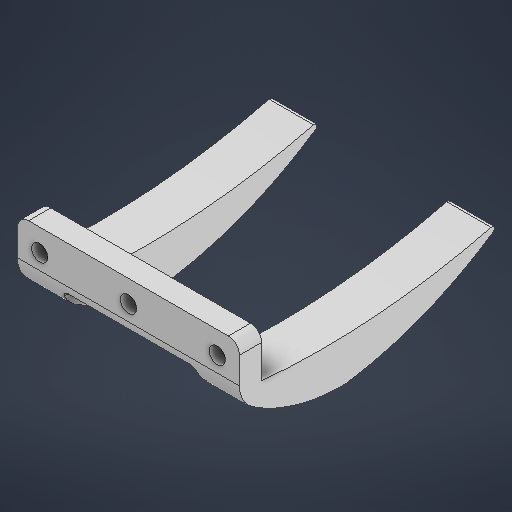
# Autodesk Inventor part: Second Stage Compression
Saved by Autodesk Inventor 2025 (Build 290162000, 162)
## iProperties
Created: 2024-12-29
Part Number: Second Stage Compression
Material: Generic
Document SubType Name: Modeling
Designer: Juan
Density: 1 g/cm^3
Appearance: Default
Author: Juan
Autodesk Inventor part; units mm, degrees
ref_plane "YZ Plane" through (0, 0, 0) normal (1, 0, 0) x (0, 1, 0)
ref_plane "XZ Plane" through (0, 0, 0) normal (0, 1, 0) x (-1, 0, 0)
ref_plane "XY Plane" through (0, 0, 0) normal (0, 0, 1) x (1, 0, 0)
sketch "Sketch1" plane through (0, 0, 0) normal (0, 0, 1) x (1, 0, 0)
  circle A0 centre (0, 0) radius 2.3241
  line L0 (0, 0) -> (12.7, 0)
  line L1 (12.7, 0) -> (25.4, 0)
  line L2 (0, 0) -> (-12.7, 0)
  line L3 (-12.7, 0) -> (-25.4, 0)
  circle A1 centre (-25.4, 0) radius 2.3241
  circle A2 centre (25.4, 0) radius 2.3241
  line L4 (-25.4, 0) -> (-31.75, 0)
  line L5 (25.4, 0) -> (31.75, 0)
  line L6 (-31.75, 6.35) -> (31.75, 6.35)
  line L7 (31.75, 6.35) -> (31.75, -6.35)
  line L8 (31.75, -6.35) -> (-31.75, -6.35)
  line L9 (-31.75, -6.35) -> (-31.75, 6.35)
  line L10 (-31.75, 6.35) -> (31.75, -6.35) construction
  line L11 (31.75, 6.35) -> (-31.75, -6.35) construction
  dimension "d0" = 4.6482
  dimension "d1" = 12.7
  dimension "d2" = 12.7
  dimension "d3" = 12.7
  dimension "d4" = 12.7
  dimension "d5" = 4.6482
  dimension "d6" = 4.6482
  dimension "d7" = 6.35
  dimension "d8" = 6.35
  dimension "d9" = 12.7
  constraints: 24 end point, 5 horizontal, 3 centre point, 3 coincident, 2 midpoint, 2 parallel, 2 point on line, 1 perpendicular
  measures "d0" diameter of A0
  measures "d1" distance of L0.start L0.end
  measures "d2" distance of L0.end L1.end
  measures "d3" distance of L0.start L2.end
  measures "d4" distance of L2.end L3.end
  measures "d5" diameter of A1
  measures "d6" diameter of A2
  measures "d7" distance of L4.start L4.end
  measures "d8" distance of L5.start L5.end
  measures "d9" distance of L6.end L7.end
extrude "Extrusion1" add sketch "Sketch1" along normal blind 6.35 contours L0 L1 A2 L5 L7 L8 L9 L4 A1 L3 L2 A0 | A0 L2 L3 A1 L4 L9 L6 L7 L5 A2 L1 L0
sketch "Sketch2" plane through (-31.75, -6.35, 0) normal (0, -1, 0) x (1, 0, 0)
  line L0 (0, 0) -> (63.5, 0) projected
  line L1 (63.5, 0) -> (63.5, 6.35) projected
  line L2 (0, 6.35) -> (63.5, 6.35) projected
  line L3 (0, 0) -> (0, 6.35) projected
  line L4 (0, 6.35) -> (63.5, 6.35)
  line L5 (63.5, 6.35) -> (63.5, -69.85)
  line L6 (63.5, -69.85) -> (0, -69.85)
  line L7 (0, -69.85) -> (0, 6.35)
  point P0 (31.75, 0)
  dimension "d12" = 76.2
  constraints: 8 end point, 2 parallel, 1 horizontal, 1 perpendicular, 1 point on line
  measures "d12" distance of L6.end L2.start
extrude "Extrusion2" add sketch "Sketch2" along normal blind 12.7
sketch "Sketch3" plane through (-31.75, 6.35, 0) normal (-1, 0, 0) x (0, 0, 1)
  line L0 (0, 0) -> (0, -12.7) projected
  line L1 (0, -12.7) -> (-69.85, -12.7) projected
  line L2 (-69.85, -12.7) -> (-69.85, -25.4) projected
  line L3 (6.35, -25.4) -> (-69.85, -25.4) projected
  line L4 (6.35, 0) -> (6.35, -25.4) projected
  line L5 (0, 0) -> (6.35, 0) projected
  line L6 (-69.85, -25.4) -> (-69.85, -6.35)
  arc A0 (-69.85, -6.35) -> (0, -12.7) centre (-17.4625, 182.5625) ccw
  arc A1 (-69.85, -19.0164) -> (-21.6074, -25.4) centre (-23.004, 149.5285) ccw
  point P0 (0, -6.35)
  point P1 (-34.925, -12.7)
  point P2 (-24.4006, -25.4)
  constraints: 4 point on circle, 3 point on line, 2 centre point, 2 end point
extrude "Extrusion3" add sketch "Sketch3" against normal up to surface (63.5 mm away) contours L1 L6 A0
extrude "Extrusion4" cut sketch "Sketch3" against normal through all contours A0 L1 | A1 L3 L2
sketch "Sketch4" plane through (-31.75, 6.35, 0) normal (-1, 0, 0) x (0, 0, 1)
  line L0 (-69.85, -6.35) -> (-69.85, -19.0164) projected
  arc A0 (-69.85, -19.0164) -> (-24.4006, -25.4) centre (-23.004, 149.5285) ccw projected
  arc A1 (-69.85, -6.35) -> (-24.4006, -25.4) centre (-8.5972, 76.0453) ccw
  point P0 (0, -6.35)
  constraints: 2 point on circle, 1 centre point
extrude "Extrusion5" cut sketch "Sketch4" against normal through all
fillet "Fillet1" radius 12.7 1 edges at (0, -19.05, -24.4006)
sketch "Sketch5" plane through (-31.75, -19.05, 0) normal (0, -1, 0) x (1, 0, 0)
  line L0 (0, 0) -> (63.5, 0) projected
  line L1 (63.5, 0) -> (0, 0)
  line L2 (63.5, 0) -> (50.8, 0)
  line L3 (63.5, 0) -> (0, 0) projected
  line L4 (0, 0) -> (12.7, 0)
  line L5 (0, -69.85) -> (63.5, -69.85) projected
  line L6 (63.5, 0) -> (50.8, 0)
  line L7 (50.8, 0) -> (50.8, -69.85)
  line L8 (50.8, -69.85) -> (63.5, -69.85)
  line L9 (63.5, -69.85) -> (63.5, 0)
  line L10 (12.7, 0) -> (0, 0)
  line L11 (0, 0) -> (0, -69.85)
  line L12 (0, -69.85) -> (12.7, -69.85)
  line L13 (12.7, -69.85) -> (12.7, 0)
  point P0 (31.75, 0)
  dimension "d22" = 12.7
  dimension "d23" = 12.7
  constraints: 22 end point, 4 parallel, 4 point on line, 3 horizontal, 2 perpendicular
  measures "d22" distance of L0.end L2.end
  measures "d23" distance of L0.start L4.end
extrude "Extrusion6" cut sketch "Sketch5" against normal blind 25.4 contours L0 L7 L5 L13
sketch "Sketch6" plane through (-31.75, 6.35, 0) normal (-1, 0, 0) x (0, 0, 1)
  arc A0 (-25.472, -25.2273) -> (-23.3846, -25.4) centre (-23.3846, -12.7) ccw projected
  line L0 (6.35, -25.4) -> (-23.3846, -25.4) projected
  line L1 (6.35, 0) -> (6.35, -25.4) projected
  line L2 (0, 0) -> (6.35, 0) projected
  line L3 (0, 0) -> (0, -12.7) projected
  arc A1 (-69.85, -6.35) -> (0, -12.7) centre (-17.4625, 182.5625) ccw projected
  arc A2 (-69.85, -6.35) -> (-25.472, -25.2273) centre (-8.5972, 76.0453) ccw projected
  line L4 (6.35, 0) -> (6.35, -25.4) projected
  arc A3 (-23.3846, -25.4) -> (6.35, -15.0552) centre (-22.7437, 20.6644) ccw
  point P0 (0, -6.35)
  point P1 (6.35, -15.0552)
  point P2 (-22.1029, -25.4)
  constraints: 2 point on circle, 1 centre point, 1 point on line
extrude "Extrusion7" cut sketch "Sketch6" against normal through all contours A3 L1 L0
fillet "Fillet2" radius 8.4667 1 edges at (0, -8.7052, 6.35)
fillet "Fillet3" radius 0.7937 2 edges at (-25.4, 0, -69.85) (25.4, 0, -69.85)
sketch "Sketch7" plane through (0, 0, 0) normal (0, 0, -1) x (-1, 0, 0)
  line L0 (-19.05, -13.0488) -> (19.05, -13.0488) projected
  line L1 (19.05, -13.0488) -> (19.05, -6.35) projected
  line L2 (31.75, -6.35) -> (19.05, -6.35) projected
  line L3 (31.75, 6.35) -> (31.75, -6.35) projected
  line L4 (-31.75, 6.35) -> (31.75, 6.35) projected
  line L5 (-31.75, -6.35) -> (-31.75, 6.35) projected
  line L6 (-19.05, -6.35) -> (-31.75, -6.35) projected
  line L7 (-19.05, -13.0488) -> (-19.05, -6.35) projected
  circle A0 centre (25.4, 0) radius 2.3241 projected
  circle A1 centre (0, 0) radius 2.3241 projected
  circle A2 centre (-25.4, 0) radius 2.3241 projected
  line L8 (19.05, -6.35) -> (-19.05, -6.35)
  constraints: 2 end point, 1 horizontal
extrude "Extrusion8" cut sketch "Sketch7" against normal blind 25.4 contours L7 L8 L1 L0
fillet "Fillet4" radius 1.5875 2 edges at (-19.05, -6.35, 3.0642) (19.05, -6.35, 3.0642)
fillet "Fillet5" radius 0.7937 2 edges at (-19.05, -7.1437, 0) (19.05, -7.1437, 0)
fillet "Fillet6" radius 3.175 2 edges at (31.75, 6.35, 3.175) (-31.75, 6.35, 3.175)
sketch "Sketch8" plane through (0, 0, 0) normal (0, 0, -1) x (-1, 0, 0)
  circle A0 centre (-25.4, 0) radius 2.3241 projected
  circle A1 centre (25.4, 0) radius 2.3241 projected
  circle A2 centre (0, 0) radius 2.3241 projected
  line L0 (-25.4, 0) -> (-12.7, 0)
  line L1 (25.4, 0) -> (12.7, 0)
  line L2 (14.8844, 2.1844) -> (10.5156, 2.1844)
  line L3 (10.5156, 2.1844) -> (10.5156, -2.1844)
  line L4 (10.5156, -2.1844) -> (14.8844, -2.1844)
  line L5 (14.8844, -2.1844) -> (14.8844, 2.1844)
  line L6 (14.8844, 2.1844) -> (10.5156, -2.1844) construction
  line L7 (10.5156, 2.1844) -> (14.8844, -2.1844) construction
  line L8 (-10.5156, 2.1844) -> (-14.8844, 2.1844)
  line L9 (-14.8844, 2.1844) -> (-14.8844, -2.1844)
  line L10 (-14.8844, -2.1844) -> (-10.5156, -2.1844)
  line L11 (-10.5156, -2.1844) -> (-10.5156, 2.1844)
  line L12 (-10.5156, 2.1844) -> (-14.8844, -2.1844) construction
  line L13 (-14.8844, 2.1844) -> (-10.5156, -2.1844) construction
  dimension "d35" = 12.7
  dimension "d36" = 12.7
  dimension "d37" = 4.3688
  dimension "d38" = 4.3688
  dimension "d39" = 4.3688
  dimension "d40" = 4.3688
  constraints: 28 end point, 4 horizontal, 4 midpoint, 4 parallel, 2 perpendicular
  measures "d35" distance of L0.start L0.end
  measures "d36" distance of L1.start L1.end
  measures "d37" distance of L4.end L3.end
  measures "d38" distance of L3.end L2.end
  measures "d39" distance of L10.end L9.end
  measures "d40" distance of L10.end L8.start
extrude "Extrusion9" add sketch "Sketch8" along normal blind 1.5875 contours L5 L4 L3 L2 | L11 L10 L9 L8
fillet "Fillet7" radius 1.016 8 edges at (10.5156, 2.1844, -0.7937) (14.8844, 2.1844, -0.7937) (14.8844, -2.1844, -0.7937) (10.5156, -2.1844, -0.7937) (-10.5156, -2.1844, -0.7937) (-14.8844, -2.1844, -0.7937) (-10.5156, 2.1844, -0.7937) (-14.8844, 2.1844, -0.7937)
body "Solid1"
